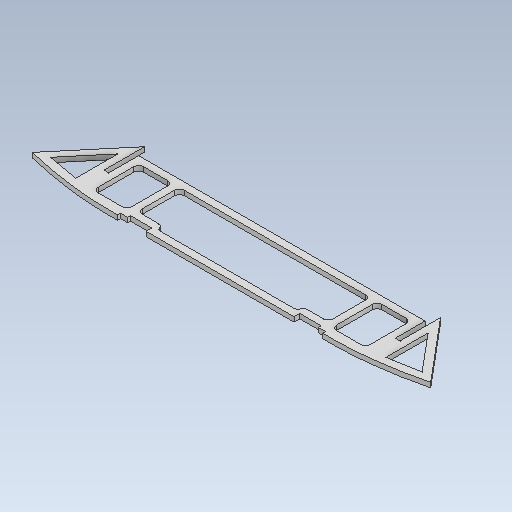
# Autodesk Inventor part: bulkhead_B2
Saved by Autodesk Inventor 2020.3 (Build 243373010, 373A)
## iProperties
Created: 2020-05-22
Part Number: bulkhead_B2
Material: Generic
Document SubType Name: Modeling
Designer: kardo
Density: 1 g/cm^3
Appearance: Default
Mass: 2.92645 g
Surface Area: 46.3053 cm^2
Volume: 2.92645 cm^3
Author: kardo
Autodesk Inventor part; units mm, degrees
ref_plane "YZ Plane" through (0, 0, 0) normal (1, 0, 0) x (0, 1, 0)
ref_plane "XZ Plane" through (0, 0, 0) normal (0, 1, 0) x (-1, 0, 0)
ref_plane "XY Plane" through (0, 0, 0) normal (0, 0, 1) x (1, 0, 0)
derived "base_sketch.ipt"
sketch "bulkhead_B2" plane through (0, -204, 0) normal (0, 1, 0) x (-1, 0, 0)
  line L0 (19.176, 46.818) -> (62.322, 46.818)
  line L1 (0, 19.935) -> (28.764, 19.935)
  line L2 (28.764, 13.529) -> (62.322, 13.529)
  line L3 (28.764, 19.935) -> (28.764, 13.529)
  line L4 (62.322, 46.818) -> (62.322, 13.529)
  line L5 (0, 9.5169) -> (0, 14.025)
  line L6 (0, 14.025) -> (62.322, 14.025)
  line L7 (0, 9.5169) -> (-21.5727, 35.2262)
  line L8 (62.322, 40.0294) -> (19.176, 40.0294)
  line L9 (-8.1416, 37.9841) -> (-8.1416, 44.7727) construction
  line L10 (-21.5727, 42.0148) -> (-21.5727, 35.2262) construction
  line L11 (19.176, 46.818) -> (19.176, 40.0294) construction
  line L12 (5.4704, 46.42) -> (5.4704, 39.6314) construction
  spline S0 degree 4 poles (-57.528, 27.54) (-46.0483, 34.2051) (-30.6129, 40.5281) (-11.2214, 45.0414) (8.3201, 46.818) (15.5662, 46.818) (19.176, 46.818) knots 0 0 0 0 0 0.630279 0.815816 1 1 1 1 1
  spline S1 degree 3 poles (19.176, 40.0294) (5.4528, 40.3024) (-8.2611, 38.4931) (-21.5727, 35.2262) knots 0 0 0 0 1 1 1 1
  line L13 (0, 45.9) -> (0, 39.1114) construction
  line L14 (-21.5727, 42.0148) -> (-8.1416, 44.7727) construction
  line L15 (-8.1416, 44.7727) -> (5.4704, 46.42) construction
  line L16 (5.4704, 46.42) -> (19.176, 46.818) construction
  point P0 (0, 0)
  point P1 (0, 7.65)
  point P2 (-38.352, 29.9314)
  point P3 (-19.176, 42.5952)
  point P4 (-38.352, 36.72)
  point P5 (0, 7.65)
ref_plane "bulkhead_B2_plane" through (0, -204, 0) normal (0, 1, 0) x (-1, 0, 0)
sketch "Sketch2" plane through (0, -204, 0) normal (0, 1, 0) x (-1, 0, 0)
  spline S0 degree 3 poles (19.176, 40.0294) (5.4528, 40.3024) (-8.2611, 38.4931) (-21.5727, 35.2262) knots 0 0 0 0 1 1 1 1 projected
  line L0 (62.322, 40.0294) -> (19.176, 40.0294) projected
  line L1 (62.322, 46.818) -> (62.322, 13.529) projected
  line L2 (0, 14.025) -> (62.322, 14.025) projected
  line L3 (0, 7.65) -> (0, 14.025) projected
  line L4 (0, 9.5169) -> (-21.5727, 35.2262) projected
  line L5 (-3, 17.7593) -> (-3, 35.5247)
  line L6 (-3, 35.5247) -> (-15.9489, 33.1913)
  line L7 (-15.9489, 33.1913) -> (-3, 17.7593)
  line L8 (7, 36.1136) -> (17.176, 36.1136)
  line L9 (19.176, 34.1136) -> (19.176, 19.025)
  line L10 (17.176, 17.025) -> (7, 17.025)
  line L11 (5, 19.025) -> (5, 34.1136)
  line L12 (62.322, 17.025) -> (24.176, 17.025)
  line L13 (22.176, 19.025) -> (22.176, 32.6294)
  line L14 (0, 14.025) -> (0, 26.5693)
  line L15 (0, 26.5693) -> (2, 26.5693)
  line L16 (2, 26.5693) -> (2, 14.025)
  line L17 (-21.5727, 35.2262) -> (0, 39.1136) construction
  line L18 (0, 39.1136) -> (0, 26.5693) construction
  arc A0 (7, 36.1136) -> (5, 34.1136) centre (7, 34.1136) ccw
  arc A1 (19.176, 34.1136) -> (17.176, 36.1136) centre (17.176, 34.1136) ccw
  arc A2 (17.176, 17.025) -> (19.176, 19.025) centre (17.176, 19.025) ccw
  arc A3 (5, 19.025) -> (7, 17.025) centre (7, 19.025) ccw
  arc A4 (22.176, 19.025) -> (24.176, 17.025) centre (24.176, 19.025) ccw
  arc A5 (24.176, 34.6294) -> (22.176, 32.6294) centre (24.176, 32.6294) ccw
  line L19 (62.322, 37.0294) -> (34.0605, 37.0294)
  line L20 (34.0605, 37.0294) -> (33.1778, 37.0294) construction
  line L21 (33.1778, 37.0294) -> (32.8048, 36.2294) construction
  line L22 (32.8048, 36.2294) -> (32.4317, 35.4294)
  line L23 (32.4317, 35.4294) -> (32.0587, 34.6294) construction
  line L24 (32.0587, 34.6294) -> (31.176, 34.6294) construction
  line L25 (31.176, 34.6294) -> (24.176, 34.6294)
  spline S1 degree 3 poles (31.176, 34.6294) (31.7112, 34.6294) (32.2056, 34.9444) (32.4317, 35.4294) knots 0 0 0 0 1 1 1 1
  spline S2 degree 3 poles (32.8048, 36.2294) (33.031, 36.7144) (33.5254, 37.0294) (34.0605, 37.0294) knots 0 0 0 0 1 1 1 1
  line L26 (19.176, 40.0294) -> (19.176, 38.8294)
  line L27 (19.176, 38.8294) -> (22.176, 38.8294)
  line L28 (22.176, 38.8294) -> (25.176, 38.8294) construction
  line L29 (25.176, 38.8294) -> (25.176, 40.0294) construction
  line L30 (22.176, 38.8294) -> (22.176, 37.6294)
  line L31 (22.176, 37.6294) -> (31.176, 37.6294)
  line L32 (31.176, 37.6294) -> (31.176, 40.0294)
  point P0 (0, 0)
  point P1 (-38.352, 29.9314)
  dimension "d1" = 3
  dimension "d2" = 3
  dimension "d3" = 3
  dimension "d4" = 2
  dimension "d5" = 3
  dimension "d6" = 3
  dimension "d10" = 3
  dimension "d11" = 3
  dimension "d12" = 2
  dimension "d15" = 3
  dimension "d16" = 3
  dimension "d17" = 115
  dimension "d18" = 1.2
  dimension "d19" = 1.2
  dimension "d20" = 6
  dimension "d22" = 6
  dimension "d23" = 3
  constraints: 56 end point, 14 parallel, 12 point on circle, 12 tangent, 8 point on line, 6 centre point, 6 equal length, 5 collinear, 5 equal radius, 5 perpendicular, 2 horizontal, 1 vertical, 9 other
  measures "d2" distance between parallel lines of L17 L6
  measures "d3" distance between parallel lines of L18 L5
  measures "d4" distance between parallel lines of L16 L14
  measures "d5" distance between parallel lines of L16 L11
  measures "d6" distance between parallel lines of L2 L10
  measures "d10" distance between parallel lines of L2 L12
  measures "d11" distance from line of L17.end L8
  measures "d12" radius of A0
  measures "d15" distance between parallel lines of L13 L9
  measures "d16" distance between parallel lines of L0 L19
  measures "d17" angle of L25 L22
  measures "d18" distance of L27.end L30.end
  measures "d19" distance of L0.end L26.end
  measures "d20" distance between parallel lines of L29 L26
  measures "d22" distance between parallel lines of L32 L29
  measures "d23" distance between parallel lines of L31 L25
extrude "Extrusion1" add sketch "Sketch2" along normal blind 2 contours L26 L27 L30 L31 L32 L0 L1 L19 S2 L22 S1 L25 A5 L13 A4 L12 L2 L16 L15 L14 L3 L4 S0
mirror "Mirror1" about plane through (-62.322, -204, 37.0294) normal (-1, 0, 0) of "Extrusion1"
equation "\"d4\" = stringer_thickness"
equation "\"d18\" = decking_thickness"
equation "\"d19\" = decking_thickness"
equation "\"d20\" = cowl_strip_width"
equation "\"d22\" = cowl_insulation_width"
equation "\"d13\" = bulkhead_thickness"
equation "\"stringer_thickness\" = 2"
equation "\"decking_thickness\" = 1.2"
equation "\"cowl_strip_width\" = 6"
equation "\"cowl_insulation_width\" = 6"
equation "\"bulkhead_thickness\" = 2"
body "Solid1"
